Autodesk Inventor part; units mm, degrees
(part 2 of 3)
  line L635 (-116.0152, 0.9815) -> (-115.9907, 0.6998)
  line L636 (-115.9907, 0.6998) -> (-115.9907, 0.6019)
  line L637 (-115.9907, 0.6019) -> (-116.1009, 0.4794)
  line L638 (-116.1009, 0.4794) -> (-116.2968, -0.4267)
  spline S120 degree 2 poles (-116.2968, -0.4267) (-116.4682, -0.7573) (-116.4805, -0.7818) knots 0 0 0 1 1 1
  line L639 (-116.4805, -0.7818) -> (-116.4438, -0.892)
  line L640 (-116.4438, -0.892) -> (-116.4438, -0.99)
  spline S121 degree 2 poles (-116.4438, -0.99) (-116.5785, -1.3083) (-116.5785, -1.4553) knots 0 0 0 1 1 1
  line L641 (-116.5785, -1.4553) -> (-116.5785, -1.6267)
  line L642 (-116.5785, -1.6267) -> (-116.6519, -1.7002)
  line L643 (-116.6519, -1.7002) -> (-116.6274, -1.9083)
  line L644 (-116.6274, -1.9083) -> (-116.6887, -1.9451)
  line L645 (-116.6887, -1.9451) -> (-116.6519, -2.092)
  line L646 (-116.6519, -2.092) -> (-116.6887, -2.1287)
  line L647 (-116.6887, -2.1287) -> (-116.6887, -2.043)
  line L648 (-116.6887, -2.043) -> (-116.7621, -2.2879)
  spline S122 degree 2 poles (-116.7621, -2.2879) (-116.8356, -2.6185) (-116.958, -2.9736) (-117.154, -3.1818) knots 0 0 0 1 2 2 2
  line L649 (-117.154, -3.1818) -> (-117.1907, -3.3165)
  line L650 (-117.1907, -3.3165) -> (-117.2519, -3.3165)
  line L651 (-117.2519, -3.3165) -> (-117.3009, -3.4267)
  line L652 (-117.3009, -3.4267) -> (-117.2519, -3.4634)
  line L653 (-117.2519, -3.4634) -> (-117.3499, -3.5369)
  line L654 (-117.3499, -3.5369) -> (-117.3254, -3.5981)
  line L655 (-117.3254, -3.5981) -> (-117.4968, -3.9287)
  line L656 (-117.4968, -3.9287) -> (-117.5336, -4.0389)
  spline S123 degree 2 poles (-117.5336, -4.0389) (-117.5458, -4.1002) (-117.7785, -4.3818) knots 0 0 0 1 1 1
  line L657 (-117.7785, -4.3818) -> (-117.7785, -4.5165)
  line L658 (-117.7785, -4.5165) -> (-117.8274, -4.4553)
  spline S124 degree 2 poles (-117.8274, -4.4553) (-118.0111, -4.6757) (-118.1091, -4.7002) knots 0 0 0 1 1 1
  line L659 (-118.1091, -4.7002) -> (-118.1091, -4.9818)
  line L660 (-118.1091, -4.9818) -> (-118.3785, -5.4838)
  line L661 (-118.3785, -5.4838) -> (-118.4887, -5.4349)
  spline S125 degree 2 poles (-118.4887, -5.4349) (-118.5744, -5.6308) (-118.7703, -5.9614) knots 0 0 0 1 1 1
  line L662 (-118.7703, -5.9614) -> (-118.9295, -6.1328)
  spline S126 degree 2 poles (-118.9295, -6.1328) (-118.9785, -6.1818) (-119.1131, -6.4879) knots 0 0 0 1 1 1
  line L663 (-119.1131, -6.4879) -> (-119.3948, -6.6104)
  line L664 (-119.3948, -6.6104) -> (-119.3948, -6.6961)
  line L665 (-119.3948, -6.6961) -> (-119.456, -6.7818)
  line L666 (-119.456, -6.7818) -> (-119.5295, -6.7206)
  line L667 (-119.5295, -6.7206) -> (-119.7499, -7.1124)
  line L668 (-119.7499, -7.1124) -> (-119.9336, -7.0022)
  line L669 (-119.9336, -7.0022) -> (-120.1417, -7.2104)
  line L670 (-120.1417, -7.2104) -> (-120.1417, -7.1736)
  line L671 (-120.1417, -7.1736) -> (-120.2152, -7.2838)
  line L672 (-120.2152, -7.2838) -> (-120.2764, -7.2838)
  line L673 (-120.2764, -7.2838) -> (-120.3254, -7.3573)
  line L674 (-120.3254, -7.3573) -> (-120.3866, -7.3941)
  line L675 (-120.3866, -7.3941) -> (-120.4356, -7.492)
  line L676 (-120.4356, -7.492) -> (-120.4968, -7.4675)
  line L677 (-120.4968, -7.4675) -> (-120.607, -7.6145)
  line L678 (-120.607, -7.6145) -> (-120.7417, -7.6145)
  line L679 (-120.7417, -7.6145) -> (-120.8274, -7.7492)
  line L680 (-120.8274, -7.7492) -> (-120.9866, -7.7492)
  line L681 (-120.9866, -7.7492) -> (-121.1336, -7.7369)
  line L682 (-121.1336, -7.7369) -> (-121.2315, -7.6512)
  spline S127 degree 2 poles (-121.2315, -7.6512) (-121.2682, -7.6145) (-121.354, -7.3941) knots 0 0 0 1 1 1
  line L683 (-121.354, -7.3941) -> (-121.1948, -7.1369)
  line L684 (-121.1948, -7.1369) -> (-120.9621, -7.0389)
  line L685 (-120.9621, -7.0389) -> (-120.8519, -6.8553)
  line L686 (-120.8519, -6.8553) -> (-120.5703, -6.8308)
  line L687 (-120.5703, -6.8308) -> (-120.4968, -6.6471)
  line L688 (-120.4968, -6.6471) -> (-120.2764, -6.6104)
  line L689 (-120.2764, -6.6104) -> (-120.1172, -6.4389)
  spline S128 degree 2 poles (-120.1172, -6.4389) (-120.0438, -6.3655) (-119.6887, -6.1573) knots 0 0 0 1 1 1
  line L690 (-119.6887, -6.1573) -> (-119.6397, -5.8634)
  line L691 (-102.9131, 8.4998) -> (-102.6805, 8.2182)
  spline S129 degree 2 poles (-102.6805, 8.2182) (-102.8519, 7.8876) (-102.9621, 7.6182) knots 0 0 0 1 1 1
  line L692 (-102.9621, 7.6182) -> (-103.2315, 7.4468)
  line L693 (-103.2315, 7.4468) -> (-103.2927, 7.2753)
  line L694 (-103.2927, 7.2753) -> (-103.2315, 7.2264)
  line L695 (-103.2315, 7.2264) -> (-103.2315, 7.0917)
  line L696 (-103.2315, 7.0917) -> (-103.207, 7.0304)
  line L697 (-103.207, 7.0304) -> (-103.2682, 6.9447)
  line L698 (-103.2682, 6.9447) -> (-103.2682, 6.7855)
  line L699 (-103.2682, 6.7855) -> (-103.3785, 6.5284)
  line L700 (-103.3785, 6.5284) -> (-103.4764, 6.4549)
  spline S130 degree 2 poles (-103.4764, 6.4549) (-103.5989, 6.1243) (-103.6601, 5.8917) knots 0 0 0 1 1 1
  line L701 (-103.6601, 5.8917) -> (-103.8193, 5.757)
  line L702 (-103.8193, 5.757) -> (-103.8805, 5.5121)
  line L703 (-103.8805, 5.5121) -> (-103.8193, 5.4753)
  line L704 (-103.8193, 5.4753) -> (-104.0152, 5.2549)
  line L705 (-104.0152, 5.2549) -> (-104.0152, 5.0957)
  line L706 (-104.0152, 5.0957) -> (-104.0764, 5.01)
  line L707 (-104.0764, 5.01) -> (-103.9785, 4.5937)
  line L708 (-103.9785, 4.5937) -> (-104.0764, 4.2386)
  line L709 (-104.0764, 4.2386) -> (-104.0152, 3.81)
  line L710 (-104.0152, 3.81) -> (-103.9295, 3.5039)
  line L711 (-103.9295, 3.5039) -> (-103.9295, 3.2223)
  line L712 (-103.9295, 3.2223) -> (-103.8805, 2.8672)
  line L713 (-103.8805, 2.8672) -> (-103.9295, 2.7202)
  line L714 (-103.9295, 2.7202) -> (-103.9295, 2.3039)
  spline S131 degree 2 poles (-103.9295, 2.3039) (-103.7213, 2.4019) (-103.6234, 2.5121) knots 0 0 0 1 1 1
  line L715 (-103.6234, 2.5121) -> (-103.4764, 2.4753)
  line L716 (-103.4764, 2.4753) -> (-103.4764, 2.5855)
  line L717 (-103.4764, 2.5855) -> (-103.1213, 2.9284)
  line L718 (-103.1213, 2.9284) -> (-102.9621, 3.0386)
  line L719 (-102.9621, 3.0386) -> (-102.9621, 3.1121)
  line L720 (-102.9621, 3.1121) -> (-102.6805, 3.357)
  line L721 (-102.6805, 3.357) -> (-102.5948, 3.6141)
  spline S132 degree 2 poles (-102.5948, 3.6141) (-102.4234, 3.6998) (-102.3131, 3.81) knots 0 0 0 1 1 1
  line L722 (-102.3131, 3.81) -> (-102.2887, 3.7611)
  line L723 (-102.2887, 3.7611) -> (-102.2887, 3.8957)
  line L724 (-102.2887, 3.8957) -> (-102.1295, 4.0304)
  line L725 (-102.1295, 4.0304) -> (-102.1295, 3.957)
  line L726 (-102.1295, 3.957) -> (-102.0682, 4.0549)
  line L727 (-102.0682, 4.0549) -> (-101.958, 4.0549)
  line L728 (-101.958, 4.0549) -> (-101.958, 4.1406)
  line L729 (-101.958, 4.1406) -> (-101.9336, 4.2019)
  line L730 (-101.9336, 4.2019) -> (-101.7866, 4.2019)
  line L731 (-101.7866, 4.2019) -> (-101.7621, 4.3121)
  line L732 (-101.7621, 4.3121) -> (-101.7866, 4.4835)
  line L733 (-101.7866, 4.4835) -> (-101.2601, 4.9121)
  spline S133 degree 2 poles (-101.2601, 4.9121) (-101.1866, 4.9733) (-101.1621, 5.0468) knots 0 0 0 1 1 1
  line L734 (-101.1621, 5.0468) -> (-101.0764, 5.2304)
  spline S134 degree 2 poles (-101.0764, 5.2304) (-100.9295, 5.3162) (-100.7948, 5.3284) knots 0 0 0 1 1 1
  line L735 (-100.7948, 5.3284) -> (-100.758, 5.4508)
  line L736 (-100.758, 5.4508) -> (-100.6846, 5.5121)
  line L737 (-100.6846, 5.5121) -> (-100.5866, 5.5121)
  line L738 (-100.5866, 5.5121) -> (-100.5866, 5.6468)
  line L739 (-100.5866, 5.6468) -> (-100.5499, 5.5366)
  line L740 (-100.5499, 5.5366) -> (-100.5499, 5.6713)
  spline S135 degree 2 poles (-100.5499, 5.6713) (-100.4764, 5.8059) (-100.4029, 5.8304) knots 0 0 0 1 1 1
  line L741 (-100.4029, 5.8304) -> (-100.3785, 5.9284)
  line L742 (-100.3785, 5.9284) -> (-100.0234, 6.308)
  line L743 (-100.0234, 6.308) -> (-99.8764, 6.308)
  line L744 (-99.8764, 6.308) -> (-99.7417, 6.4549)
  line L745 (-99.7417, 6.4549) -> (-99.5948, 6.7488)
  spline S136 degree 2 poles (-99.5948, 6.7488) (-99.2274, 7.1529) (-99.1785, 7.2753) knots 0 0 0 1 1 1
  line L746 (-99.1785, 7.2753) -> (-98.958, 7.3121)
  line L747 (-98.958, 7.3121) -> (-98.7621, 7.6672)
  line L748 (-98.7621, 7.6672) -> (-98.8234, 7.4835)
  line L749 (-98.8234, 7.4835) -> (-98.5417, 7.7039)
  line L750 (-98.5417, 7.7039) -> (-98.3703, 7.5815)
  line L751 (-98.3703, 7.5815) -> (-98.1499, 7.7284)
  line L752 (-98.1499, 7.7284) -> (-97.8682, 7.7284)
  line L753 (-97.8682, 7.7284) -> (-97.7336, 7.6182)
  line L754 (-97.7336, 7.6182) -> (-97.6846, 7.3488)
  line L755 (-97.6846, 7.3488) -> (-97.807, 7.2264)
  spline S137 degree 2 poles (-97.807, 7.2264) (-97.8682, 7.1651) (-97.9785, 6.9202) knots 0 0 0 1 1 1
  line L756 (-97.9785, 6.9202) -> (-97.9295, 6.7855)
  line L757 (-97.9295, 6.7855) -> (-98.0152, 6.5284)
  line L758 (-98.0152, 6.5284) -> (-98.0152, 6.4304)
  line L759 (-98.0152, 6.4304) -> (-98.1254, 6.308)
  line L760 (-98.1254, 6.308) -> (-98.1254, 6.1121)
  line L761 (-98.1254, 6.1121) -> (-98.2601, 6.0753)
  line L762 (-98.2601, 6.0753) -> (-98.2601, 5.6713)
  line L763 (-98.2601, 5.6713) -> (-98.2846, 5.5121)
  line L764 (-98.2846, 5.5121) -> (-98.2601, 5.3284)
  line L765 (-98.2601, 5.3284) -> (-98.407, 5.1937)
  line L766 (-98.407, 5.1937) -> (-98.3213, 5.01)
  line L767 (-98.3213, 5.01) -> (-98.407, 4.8753)
  line L768 (-98.407, 4.8753) -> (-98.3213, 4.5325)
  line L769 (-98.3213, 4.5325) -> (-98.407, 4.3366)
  line L770 (-98.407, 4.3366) -> (-98.407, 3.0019)
  line L771 (-98.407, 3.0019) -> (-98.3213, 2.7202)
  line L772 (-98.3213, 2.7202) -> (-98.1866, 2.6223)
  line L773 (-98.1866, 2.6223) -> (-97.905, 2.6468)
  line L774 (-97.905, 2.6468) -> (-97.7703, 2.5121)
  line L775 (-97.7703, 2.5121) -> (-97.7948, 2.3406)
  line L776 (-97.7948, 2.3406) -> (-97.9785, 2.2549)
  line L777 (-97.9785, 2.2549) -> (-98.0519, 2.0835)
  line L778 (-98.0519, 2.0835) -> (-98.1866, 2.059)
  line L779 (-98.1866, 2.059) -> (-98.2846, 1.8753)
  line L780 (-98.2846, 1.8753) -> (-98.407, 1.8753)
  line L781 (-98.407, 1.8753) -> (-98.4682, 1.7039)
  line L782 (-98.4682, 1.7039) -> (-98.7866, 1.5937)
  line L783 (-98.7866, 1.5937) -> (-98.8968, 1.3855)
  line L784 (-98.8968, 1.3855) -> (-99.3254, 1.3121)
  line L785 (-99.3254, 1.3121) -> (-99.4846, 1.1406)
  line L786 (-99.4846, 1.1406) -> (-99.8397, 1.0672)
  line L787 (-99.8397, 1.0672) -> (-100.0234, 1.1774)
  line L788 (-100.0234, 1.1774) -> (-100.158, 1.6182)
  line L789 (-100.158, 1.6182) -> (-100.0234, 1.8141)
  line L790 (-100.0234, 1.8141) -> (-100.0968, 1.9488)
  line L791 (-100.0968, 1.9488) -> (-99.9866, 2.0835)
  line L792 (-99.9866, 2.0835) -> (-99.8397, 2.1202)
  line L793 (-99.8397, 2.1202) -> (-99.6805, 3.1733)
  line L794 (-99.6805, 3.1733) -> (-99.6805, 3.3202)
  line L795 (-99.6805, 3.3202) -> (-99.7662, 3.5039)
  line L796 (-99.7662, 3.5039) -> (-99.6315, 3.5651)
  line L797 (-99.6315, 3.5651) -> (-99.6805, 3.6998)
  line L798 (-99.6805, 3.6998) -> (-99.6315, 3.8957)
  line L799 (-99.6315, 3.8957) -> (-99.7662, 3.957)
  line L800 (-99.7662, 3.957) -> (-99.8397, 4.0549)
  line L801 (-99.8397, 4.0549) -> (-99.705, 4.1774)
  line L802 (-99.705, 4.1774) -> (-99.705, 4.3366)
  line L803 (-99.705, 4.3366) -> (-99.6315, 4.5325)
  spline S138 degree 2 poles (-99.6315, 4.5325) (-99.8274, 4.6917) (-99.9009, 4.6917) knots 0 0 0 1 1 1
  line L804 (-99.9009, 4.6917) -> (-99.9499, 5.059)
  line L805 (-99.9499, 5.059) -> (-100.0968, 5.059)
  line L806 (-100.0968, 5.059) -> (-100.207, 5.1202)
  line L807 (-100.207, 5.1202) -> (-100.3417, 4.8753)
  line L808 (-100.3417, 4.8753) -> (-101.1254, 4.0304)
  line L809 (-101.1254, 4.0304) -> (-101.2601, 3.9202)
  line L810 (-101.2601, 3.9202) -> (-101.2968, 3.81)
  line L811 (-101.2968, 3.81) -> (-101.8968, 3.1121)
  line L812 (-101.8968, 3.1121) -> (-101.958, 2.9774)
  line L813 (-101.958, 2.9774) -> (-102.5948, 2.2304)
  line L814 (-102.5948, 2.2304) -> (-103.3785, 1.3855)
  line L815 (-103.3785, 1.3855) -> (-103.6111, 1.2631)
  spline S139 degree 2 poles (-103.6111, 1.2631) (-103.6601, 1.2386) (-103.758, 1.0672) knots 0 0 0 1 1 1
  spline S140 degree 2 poles (-103.758, 1.0672) (-104.0887, 0.9447) (-104.1131, 0.9202) knots 0 0 0 1 1 1
  line L816 (-104.1131, 0.9202) -> (-104.1131, 0.8468)
  line L817 (-104.1131, 0.8468) -> (-104.2111, 0.8957)
  line L818 (-104.2111, 0.8957) -> (-104.2111, 0.6753)
  line L819 (-104.2111, 0.6753) -> (-104.4315, 0.5406)
  line L820 (-104.4315, 0.5406) -> (-104.7131, 0.5651)
  line L821 (-104.7131, 0.5651) -> (-104.9948, 0.3692)
  line L822 (-104.9948, 0.3692) -> (-105.0315, 0.4672)
  line L823 (-105.0315, 0.4672) -> (-105.2152, 0.5651)
  line L824 (-105.2152, 0.5651) -> (-105.2397, 0.7488)
  spline S141 degree 2 poles (-105.2397, 0.7488) (-105.3499, 0.8345) (-105.4234, 1.0059) knots 0 0 0 1 1 1
  line L825 (-105.4234, 1.0059) -> (-105.5948, 1.0672)
  line L826 (-105.5948, 1.0672) -> (-105.656, 1.2386)
  line L827 (-105.656, 1.2386) -> (-105.7662, 2.4508)
  line L828 (-105.7662, 2.4508) -> (-105.656, 2.9039)
  line L829 (-105.656, 2.9039) -> (-105.5948, 2.9039)
  line L830 (-105.5948, 2.9039) -> (-105.5948, 3.2223)
  line L831 (-105.5948, 3.2223) -> (-105.4234, 3.357)
  line L832 (-105.4234, 3.357) -> (-105.4478, 3.5039)
  line L833 (-105.4478, 3.5039) -> (-105.3499, 3.7611)
  line L834 (-105.3499, 3.7611) -> (-105.2152, 3.7611)
  line L835 (-105.2152, 3.7611) -> (-105.1785, 3.8468)
  line L836 (-105.1785, 3.8468) -> (-105.2152, 4.0549)
  line L837 (-105.2152, 4.0549) -> (-105.0927, 4.0917)
  line L838 (-105.0927, 4.0917) -> (-105.0682, 4.3366)
  line L839 (-105.0682, 4.3366) -> (-105.0315, 4.3733)
  line L840 (-105.0315, 4.3733) -> (-105.1295, 4.4835)
  line L841 (-105.1295, 4.4835) -> (-105.0315, 4.6917)
  line L842 (-105.0315, 4.6917) -> (-105.0315, 4.9488)
  line L843 (-105.0315, 4.9488) -> (-104.9948, 5.4753)
  line L844 (-104.9948, 5.4753) -> (-104.9336, 5.4753)
  line L845 (-104.9336, 5.4753) -> (-104.9336, 5.7325)
  line L846 (-104.9336, 5.7325) -> (-104.7866, 5.8917)
  line L847 (-104.7866, 5.8917) -> (-104.8968, 6.0386)
  line L848 (-104.8968, 6.0386) -> (-104.7866, 6.2223)
  line L849 (-104.7866, 6.2223) -> (-104.8234, 6.308)
  line L850 (-104.8234, 6.308) -> (-104.6764, 6.5896)
  line L851 (-104.6764, 6.5896) -> (-104.8968, 6.8468)
  line L852 (-104.8968, 6.8468) -> (-105.0315, 6.81)
  line L853 (-105.0315, 6.81) -> (-105.0682, 6.6753)
  line L854 (-105.0682, 6.6753) -> (-105.2764, 6.6386)
  line L855 (-105.2764, 6.6386) -> (-105.3499, 6.4549)
  line L856 (-105.3499, 6.4549) -> (-105.5948, 6.4549)
  line L857 (-105.5948, 6.4549) -> (-105.705, 6.5896)
  line L858 (-105.705, 6.5896) -> (-106.5499, 6.308)
  line L859 (-106.5499, 6.308) -> (-106.7703, 6.6753)
  line L860 (-106.7703, 6.6753) -> (-106.4887, 6.9447)
  spline S142 degree 2 poles (-106.4887, 6.9447) (-106.2682, 7.0427) (-106.207, 7.2264) knots 0 0 0 1 1 1
  line L861 (-106.207, 7.2264) -> (-105.9499, 7.2753)
  line L862 (-105.9499, 7.2753) -> (-105.9499, 7.3488)
  line L863 (-105.9499, 7.3488) -> (-105.7295, 7.3488)
  line L864 (-105.7295, 7.3488) -> (-105.4478, 7.3733)
  line L865 (-105.4478, 7.3733) -> (-105.2764, 7.7039)
  line L866 (-105.2764, 7.7039) -> (-104.9948, 7.6182)
  line L867 (-104.9948, 7.6182) -> (-104.6764, 7.7039)
  spline S143 degree 2 poles (-104.6764, 7.7039) (-104.6519, 7.7651) (-104.5785, 7.8264) knots 0 0 0 1 1 1
  line L868 (-104.5785, 7.8264) -> (-104.3213, 7.8264)
  line L869 (-104.3213, 7.8264) -> (-104.358, 7.8631)
  line L870 (-104.358, 7.8631) -> (-104.2968, 7.8998)
  line L871 (-104.2968, 7.8998) -> (-104.1131, 7.8998)
  line L872 (-104.1131, 7.8998) -> (-104.0764, 7.9855)
  spline S144 degree 2 poles (-104.0764, 7.9855) (-103.905, 8.0468) (-103.7336, 8.2182) knots 0 0 0 1 1 1
  line L873 (-103.7336, 8.2182) -> (-103.5989, 8.2182)
  line L874 (-103.5989, 8.2182) -> (-103.4764, 8.3651)
  line L875 (-103.4764, 8.3651) -> (-103.3785, 8.4019)
  line L876 (-103.3785, 8.4019) -> (-103.2682, 8.3651)
  line L877 (-103.2682, 8.3651) -> (-103.1213, 8.4386)
  line L878 (-103.1213, 8.4386) -> (-103.0478, 8.3651)
  line L879 (-103.0478, 8.3651) -> (-102.9866, 8.4998)
  line L880 (-102.9866, 8.4998) -> (-102.9131, 8.4998)
  line L881 (-83.9825, 12.81) -> (-83.9213, 12.7733)
  line L882 (-83.9213, 12.7733) -> (-83.7499, 12.7733)
  line L883 (-83.7499, 12.7733) -> (-83.0519, 12.2835)
  line L884 (-83.0519, 12.2835) -> (-82.5499, 11.757)
  line L885 (-82.5499, 11.757) -> (-83.3825, 11.1447)
  line L886 (-83.3825, 11.1447) -> (-83.4927, 11.01)
  line L887 (-83.4927, 11.01) -> (-84.0682, 10.8753)
  line L888 (-84.0682, 10.8753) -> (-84.3499, 10.8998)
  line L889 (-84.3499, 10.8998) -> (-84.5948, 11.0835)
  line L890 (-84.5948, 11.0835) -> (-84.7417, 11.0835)
  line L891 (-84.7417, 11.0835) -> (-85.3785, 9.7855)
  line L892 (-85.3785, 9.7855) -> (-85.6601, 9.4549)
  line L893 (-85.6601, 9.4549) -> (-85.6846, 9.1121)
  line L894 (-85.6846, 9.1121) -> (-85.9295, 8.6468)
  line L895 (-85.9295, 8.6468) -> (-86.0397, 8.2917)
  line L896 (-86.0397, 8.2917) -> (-86.1744, 8.0835)
  line L897 (-86.1744, 8.0835) -> (-86.2356, 7.5815)
  line L898 (-86.2356, 7.5815) -> (-86.3336, 7.3243)
  spline S145 degree 2 poles (-86.3336, 7.3243) (-86.358, 7.2753) (-86.5417, 7.0917) knots 0 0 0 1 1 1
  line L899 (-86.5417, 7.0917) -> (-86.5417, 6.9202)
  line L900 (-86.5417, 6.9202) -> (-86.6397, 6.5896)
  line L901 (-86.6397, 6.5896) -> (-86.5662, 6.3937)
  spline S146 degree 2 poles (-86.5662, 6.3937) (-86.6764, 6.0386) (-86.7744, 5.8917) knots 0 0 0 1 1 1
  line L902 (-86.7744, 5.8917) -> (-86.7376, 5.61)
  line L903 (-86.7376, 5.61) -> (-86.8478, 5.2549)
  line L904 (-86.8478, 5.2549) -> (-86.7744, 5.1937)
  line L905 (-86.7744, 5.1937) -> (-86.7744, 5.01)
  line L906 (-86.7744, 5.01) -> (-86.6397, 4.8753)
  line L907 (-86.6397, 4.8753) -> (-86.7131, 4.6182)
  line L908 (-86.7131, 4.6182) -> (-86.6397, 4.0549)
  line L909 (-86.6397, 4.0549) -> (-86.6764, 4.0549)
  line L910 (-86.6764, 4.0549) -> (-86.7131, 3.6386)
  spline S147 degree 2 poles (-86.7131, 3.6386) (-86.7131, 3.5162) (-86.3825, 3.1488) knots 0 0 0 1 1 1
  line L911 (-86.3825, 3.1488) -> (-86.456, 3.0386)
  line L912 (-86.456, 3.0386) -> (-86.3213, 2.8672)
  line L913 (-86.3213, 2.8672) -> (-86.2356, 2.157)
  line L914 (-86.2356, 2.157) -> (-86.4315, 1.9855)
  line L915 (-86.4315, 1.9855) -> (-86.4315, 1.7774)
  line L916 (-86.4315, 1.7774) -> (-86.5417, 1.5325)
  line L917 (-86.5417, 1.5325) -> (-86.6397, 1.5325)
  line L918 (-86.6397, 1.5325) -> (-86.958, 1.0672)
  line L919 (-86.958, 1.0672) -> (-87.2397, 1.0917)
  line L920 (-87.2397, 1.0917) -> (-87.4846, 0.7978)
  line L921 (-87.4846, 0.7978) -> (-87.9376, 0.4672)
  line L922 (-87.9376, 0.4672) -> (-88.2682, 1.0672)
  line L923 (-88.2682, 1.0672) -> (-88.2682, 1.6672)
  line L924 (-88.2682, 1.6672) -> (-88.3662, 2.2059)
  line L925 (-88.3662, 2.2059) -> (-88.3295, 2.4508)
  line L926 (-88.3295, 2.4508) -> (-88.758, 3.0753)
  line L927 (-88.758, 3.0753) -> (-88.6478, 3.259)
  line L928 (-88.6478, 3.259) -> (-88.758, 3.4549)
  line L929 (-88.758, 3.4549) -> (-88.6846, 3.5406)
  line L930 (-88.6846, 3.5406) -> (-88.9662, 3.6386)
  line L931 (-88.9662, 3.6386) -> (-89.0642, 3.5651)
  spline S148 degree 2 poles (-89.0642, 3.5651) (-89.1131, 3.6998) (-89.3458, 3.9692) knots 0 0 0 1 1 1
  line L932 (-89.3458, 3.9692) -> (-89.456, 3.9692)
  line L933 (-89.456, 3.9692) -> (-89.6274, 4.557)
  line L934 (-89.6274, 4.557) -> (-89.958, 4.8508)
  line L935 (-89.958, 4.8508) -> (-90.1295, 5.1937)
  spline S149 degree 2 poles (-90.1295, 5.1937) (-90.2519, 5.4141) (-90.2642, 5.5488) knots 0 0 0 1 1 1
  line L936 (-90.2642, 5.5488) -> (-90.6805, 5.9406)
  line L937 (-90.6805, 5.9406) -> (-90.7907, 6.1611)
  line L938 (-90.7907, 6.1611) -> (-90.7662, 6.3325)
  line L939 (-90.7662, 6.3325) -> (-90.8764, 6.5039)
  line L940 (-90.8764, 6.5039) -> (-90.9866, 6.5529)
  line L941 (-90.9866, 6.5529) -> (-91.0723, 6.7855)
  line L942 (-91.0723, 6.7855) -> (-91.158, 6.7855)
  line L943 (-91.158, 6.7855) -> (-91.2682, 7.0794)
  line L944 (-91.2682, 7.0794) -> (-91.4887, 7.3611)
  spline S150 degree 2 poles (-91.4887, 7.3611) (-91.5254, 7.4223) (-91.5744, 7.6427) knots 0 0 0 1 1 1
  line L945 (-91.5744, 7.6427) -> (-91.758, 7.6059)
  line L946 (-91.758, 7.6059) -> (-91.9662, 7.1651)
  line L947 (-91.9662, 7.1651) -> (-91.9662, 7.0304)
  spline S151 degree 2 poles (-91.9662, 7.0304) (-92.0152, 6.7243) (-92.1376, 6.3692) knots 0 0 0 1 1 1
  line L948 (-92.1376, 6.3692) -> (-92.2846, 6.2835)
  line L949 (-92.2846, 6.2835) -> (-92.2111, 6.0386)
  line L950 (-92.2111, 6.0386) -> (-92.0397, 5.9284)
  line L951 (-92.0397, 5.9284) -> (-92.1009, 5.5855)
  line L952 (-92.1009, 5.5855) -> (-92.1009, 5.1937)
  line L953 (-92.1009, 5.1937) -> (-92.456, 4.7651)
  line L954 (-92.456, 4.7651) -> (-92.4315, 4.459)
  line L955 (-92.4315, 4.459) -> (-92.5172, 4.2386)
  line L956 (-92.5172, 4.2386) -> (-92.4315, 3.9937)
  line L957 (-92.4315, 3.9937) -> (-92.4927, 3.9202)
  line L958 (-92.4927, 3.9202) -> (-92.456, 3.6998)
  line L959 (-92.456, 3.6998) -> (-92.6029, 3.3937)
  line L960 (-92.6029, 3.3937) -> (-92.6029, 3.1733)
  line L961 (-92.6029, 3.1733) -> (-92.7376, 3.0019)
  line L962 (-92.7376, 3.0019) -> (-92.8478, 2.5366)
  line L963 (-92.8478, 2.5366) -> (-92.8478, 2.4019)
  line L964 (-92.8478, 2.4019) -> (-92.9091, 2.3406)
  line L965 (-92.9091, 2.3406) -> (-93.2642, 1.2386)
  line L966 (-93.2642, 1.2386) -> (-93.3744, 1.0304)
  line L967 (-93.3744, 1.0304) -> (-93.656, 0.8957)
  line L968 (-93.656, 0.8957) -> (-93.6193, 0.81)
  line L969 (-93.6193, 0.81) -> (-94.1825, 0.5651)
  line L970 (-94.1825, 0.5651) -> (-94.4642, 0.6386)
  line L971 (-94.4642, 0.6386) -> (-94.5376, 0.9202)
  line L972 (-94.5376, 0.9202) -> (-94.354, 1.1406)
  line L973 (-94.354, 1.1406) -> (-94.4397, 1.2386)
  line L974 (-94.4397, 1.2386) -> (-94.6478, 1.2386)
  line L975 (-94.6478, 1.2386) -> (-94.6478, 1.3121)
  line L976 (-94.6478, 1.3121) -> (-94.4029, 1.5325)
  line L977 (-94.4029, 1.5325) -> (-94.4642, 1.8141)
  line L978 (-94.4642, 1.8141) -> (-94.2193, 1.8753)
  line L979 (-94.2193, 1.8753) -> (-93.8764, 2.3406)
  line L980 (-93.8764, 2.3406) -> (-93.7662, 2.757)
  line L981 (-93.7662, 2.757) -> (-93.7662, 2.9284)
  line L982 (-93.7662, 2.9284) -> (-93.5948, 3.1121)
  line L983 (-93.5948, 3.1121) -> (-93.5948, 3.4304)
  line L984 (-93.5948, 3.4304) -> (-93.1295, 5.3284)
  line L985 (-93.1295, 5.3284) -> (-93.154, 5.4508)
  line L986 (-93.154, 5.4508) -> (-93.154, 5.757)
  line L987 (-93.154, 5.757) -> (-92.958, 6.0753)
  line L988 (-92.958, 6.0753) -> (-93.0193, 6.2835)
  line L989 (-93.0193, 6.2835) -> (-92.8478, 6.5651)
  line L990 (-92.8478, 6.5651) -> (-92.8233, 6.7488)
  line L991 (-92.8233, 6.7488) -> (-92.7376, 7.0304)
  line L992 (-92.7376, 7.0304) -> (-92.7744, 7.1651)
  line L993 (-92.7744, 7.1651) -> (-92.6642, 7.5815)
  line L994 (-92.6642, 7.5815) -> (-92.958, 8.3406)
  spline S152 degree 2 poles (-92.958, 8.3406) (-92.8846, 8.4386) (-92.7376, 8.5366) knots 0 0 0 1 1 1
  line L995 (-92.7376, 8.5366) -> (-92.8478, 8.9284)
  line L996 (-92.8478, 8.9284) -> (-92.7744, 9.1733)
  line L997 (-92.7744, 9.1733) -> (-92.6274, 9.1978)
  line L998 (-92.6274, 9.1978) -> (-92.6029, 9.4182)
  line L999 (-92.6029, 9.4182) -> (-93.2397, 9.4182)
  line L1000 (-93.2397, 9.4182) -> (-93.8764, 9.1978)
  line L1001 (-93.8764, 9.1978) -> (-94.0111, 9.2835)
  line L1002 (-94.0111, 9.2835) -> (-94.354, 8.5855)
  line L1003 (-94.354, 8.5855) -> (-95.2356, 7.7651)
  line L1004 (-95.2356, 7.7651) -> (-95.7131, 7.557)
  line L1005 (-95.7131, 7.557) -> (-95.9091, 7.9488)
  line L1006 (-95.9091, 7.9488) -> (-95.9091, 8.2182)
  line L1007 (-95.9091, 8.2182) -> (-95.7376, 8.2917)
  line L1008 (-95.7376, 8.2917) -> (-95.7744, 8.4386)
  line L1009 (-95.7744, 8.4386) -> (-95.8723, 8.4753)
  line L1010 (-95.8723, 8.4753) -> (-95.8723, 8.6468)
  line L1011 (-95.8723, 8.6468) -> (-95.7131, 8.7815)
  line L1012 (-95.7131, 8.7815) -> (-95.7131, 8.9284)
  line L1013 (-95.7131, 8.9284) -> (-95.4315, 8.8304)
  line L1014 (-95.4315, 8.8304) -> (-95.358, 8.9284)
  line L1015 (-95.358, 8.9284) -> (-95.456, 9.0386)
  spline S153 degree 2 poles (-95.456, 9.0386) (-95.4315, 9.1121) (-95.1376, 9.4549) knots 0 0 0 1 1 1
  line L1016 (-95.1376, 9.4549) -> (-94.7458, 9.5651)
  line L1017 (-94.7458, 9.5651) -> (-94.7213, 9.81)
  line L1018 (-94.7213, 9.81) -> (-94.5376, 9.7855)
  line L1019 (-94.5376, 9.7855) -> (-94.3907, 9.9447)
  spline S154 degree 2 poles (-94.3907, 9.9447) (-94.354, 9.9815) (-94.2315, 10.0304) knots 0 0 0 1 1 1
  line L1020 (-94.2315, 10.0304) -> (-93.9376, 10.1406)
  line L1021 (-93.9376, 10.1406) -> (-93.9009, 10.2019)
  line L1022 (-93.9009, 10.2019) -> (-93.6927, 10.2141)
  spline S155 degree 2 poles (-93.6927, 10.2141) (-93.558, 10.2386) (-93.3621, 10.3855) (-92.9948, 10.4468) knots 0 0 0 1 2 2 2
  line L1023 (-92.9948, 10.4468) -> (-92.6274, 10.508)
  line L1024 (-92.6274, 10.508) -> (-91.7825, 10.9978)
  line L1025 (-91.7825, 10.9978) -> (-91.5744, 11.2182)
  line L1026 (-91.5744, 11.2182) -> (-91.1458, 11.3774)
  line L1027 (-91.1458, 11.3774) -> (-90.7662, 11.4264)
  line L1028 (-90.7662, 11.4264) -> (-90.5703, 11.0223)
  spline S156 degree 2 poles (-90.5703, 11.0223) (-90.7907, 10.6427) (-90.7417, 10.459) knots 0 0 0 1 1 1
  line L1029 (-90.7417, 10.459) -> (-90.5213, 9.2345)
  line L1030 (-90.5213, 9.2345) -> (-90.4111, 8.9406)
  line L1031 (-90.4111, 8.9406) -> (-90.4111, 8.7447)
  line L1032 (-90.4111, 8.7447) -> (-90.2029, 8.7447)
  line L1033 (-90.2029, 8.7447) -> (-90.1785, 8.4264)
  line L1034 (-90.1785, 8.4264) -> (-89.8478, 8.1447)
  line L1035 (-89.8478, 8.1447) -> (-89.8846, 7.9488)
  line L1036 (-89.8846, 7.9488) -> (-89.8111, 7.8631)
  line L1037 (-89.8111, 7.8631) -> (-89.2111, 6.8468)
  line L1038 (-89.2111, 6.8468) -> (-88.5744, 5.5855)
  line L1039 (-88.5744, 5.5855) -> (-88.4029, 5.4019)
  line L1040 (-88.4029, 5.4019) -> (-88.4029, 5.3039)
  line L1041 (-88.4029, 5.3039) -> (-88.2682, 5.157)
  line L1042 (-88.2682, 5.157) -> (-88.0478, 5.1202)
  line L1043 (-88.0478, 5.1202) -> (-88.0111, 5.3039)
  line L1044 (-88.0111, 5.3039) -> (-87.9131, 5.3284)
  line L1045 (-87.9131, 5.3284) -> (-87.9131, 5.4508)
  line L1046 (-87.9131, 5.4508) -> (-87.6315, 6.3692)
  line L1047 (-87.6315, 6.3692) -> (-87.607, 6.5896)
  spline S157 degree 2 poles (-87.607, 6.5896) (-87.5948, 6.6753) (-87.4601, 7.0672) knots 0 0 0 1 1 1
  line L1048 (-87.4601, 7.0672) -> (-87.154, 7.2753)
  line L1049 (-87.154, 7.2753) -> (-87.154, 7.4468)
  line L1050 (-87.154, 7.4468) -> (-86.9948, 7.7284)
  line L1051 (-86.9948, 7.7284) -> (-86.9948, 7.9488)
  spline S158 degree 2 poles (-86.9948, 7.9488) (-86.8233, 8.157) (-86.7376, 8.4998) knots 0 0 0 1 1 1
  spline S159 degree 2 poles (-86.7376, 8.4998) (-86.6887, 8.5243) (-86.6152, 8.6223) knots 0 0 0 1 1 1
  line L1052 (-86.6152, 8.6223) -> (-86.5417, 8.7202)
  line L1053 (-86.5417, 8.7202) -> (-86.1009, 9.8835)
  spline S160 degree 2 poles (-86.1009, 9.8835) (-86.0274, 10.0549) (-85.954, 10.1039) knots 0 0 0 1 1 1
  line L1054 (-85.954, 10.1039) -> (-85.856, 10.508)
  line L1055 (-85.856, 10.508) -> (-85.7213, 10.6182)
  line L1056 (-85.7213, 10.6182) -> (-85.5376, 10.9488)
  line L1057 (-85.5376, 10.9488) -> (-85.4397, 11.2549)
  line L1058 (-85.4397, 11.2549) -> (-85.305, 11.4264)
  spline S161 degree 2 poles (-85.305, 11.4264) (-85.2315, 11.4998) (-85.158, 11.7202) knots 0 0 0 1 1 1
  line L1059 (-85.158, 11.7202) -> (-85.0233, 11.757)
  line L1060 (-85.0233, 11.757) -> (-84.6193, 12.4917)
  line L1061 (-84.6193, 12.4917) -> (-84.4601, 12.6386)
  line L1062 (-84.4601, 12.6386) -> (-84.3866, 12.6386)
  spline S162 degree 2 poles (-84.3866, 12.6386) (-84.2887, 12.7733) (-84.2397, 12.7733) knots 0 0 0 1 1 1
  line L1063 (-84.2397, 12.7733) -> (-83.9825, 12.81)
  line L1064 (-79.158, 8.2182) -> (-78.9744, 8.1937)
  line L1065 (-78.9744, 8.1937) -> (-78.9376, 8.1937)
  line L1066 (-78.9376, 8.1937) -> (-78.9744, 8.1202)
  line L1067 (-78.9744, 8.1202) -> (-78.9131, 8.1202)
  line L1068 (-78.9131, 8.1202) -> (-78.8029, 8.01)
  line L1069 (-78.8029, 8.01) -> (-78.4478, 7.9855)
  line L1070 (-78.4478, 7.9855) -> (-78.0927, 7.9855)
  line L1071 (-78.0927, 7.9855) -> (-77.8846, 7.8631)
  line L1072 (-77.8846, 7.8631) -> (-77.8111, 7.8631)
  line L1073 (-77.8111, 7.8631) -> (-77.7009, 7.4835)
  line L1074 (-77.7009, 7.4835) -> (-77.8601, 7.3488)
  line L1075 (-77.8601, 7.3488) -> (-77.8601, 7.2019)
  line L1076 (-77.8601, 7.2019) -> (-77.6029, 6.9447)
  line L1077 (-77.6029, 6.9447) -> (-77.6397, 6.2468)
  line L1078 (-77.6397, 6.2468) -> (-77.7499, 6.2468)
  line L1079 (-77.7499, 6.2468) -> (-77.7866, 6.1121)
  line L1080 (-77.7866, 6.1121) -> (-77.8111, 6.1121)
  line L1081 (-77.8111, 6.1121) -> (-77.8111, 5.8917)
  line L1082 (-77.8111, 5.8917) -> (-77.6642, 5.8672)
  line L1083 (-77.6642, 5.8672) -> (-77.6029, 5.7937)
  line L1084 (-77.6029, 5.7937) -> (-77.7009, 5.6468)
  line L1085 (-77.7009, 5.6468) -> (-77.7009, 5.5366)
  line L1086 (-77.7009, 5.5366) -> (-77.8846, 5.4508)
  line L1087 (-77.8846, 5.4508) -> (-78.0193, 5.3284)
  line L1088 (-78.0193, 5.3284) -> (-78.4233, 5.1202)
  spline S163 degree 2 poles (-78.4233, 5.1202) (-78.5825, 4.9488) (-78.6927, 4.8753) knots 0 0 0 1 1 1
  line L1089 (-78.6927, 4.8753) -> (-78.8029, 4.557)
  line L1090 (-78.8029, 4.557) -> (-79.4764, 4.2998)
  line L1091 (-79.4764, 4.2998) -> (-80.1376, 4.3121)
  line L1092 (-80.1376, 4.3121) -> (-80.1131, 4.1406)
  line L1093 (-80.1131, 4.1406) -> (-80.2478, 4.1406)
  line L1094 (-80.2478, 4.1406) -> (-80.2846, 4.0917)
  line L1095 (-80.2846, 4.0917) -> (-80.6029, 4.0304)
  line L1096 (-80.6029, 4.0304) -> (-80.6397, 4.1406)
  line L1097 (-80.6397, 4.1406) -> (-80.7499, 4.0917)
  line L1098 (-80.7499, 4.0917) -> (-80.7499, 4.0304)
  line L1099 (-80.7499, 4.0304) -> (-81.0315, 3.9202)
  line L1100 (-81.0315, 3.9202) -> (-81.1417, 3.6141)
  line L1101 (-81.1417, 3.6141) -> (-80.9948, 3.2223)
  line L1102 (-80.9948, 3.2223) -> (-80.9948, 3.0386)
  line L1103 (-80.9948, 3.0386) -> (-80.9213, 2.8672)
  spline S164 degree 2 poles (-80.9213, 2.8672) (-81.0682, 2.4141) (-81.1417, 2.4019) knots 0 0 0 1 1 1
  line L1104 (-81.1417, 2.4019) -> (-81.0927, 2.2549)
  line L1105 (-81.0927, 2.2549) -> (-81.1662, 2.2304)
  line L1106 (-81.1662, 2.2304) -> (-80.9948, 2.157)
  line L1107 (-80.9948, 2.157) -> (-80.9948, 1.9243)
  line L1108 (-80.9948, 1.9243) -> (-80.8356, 1.8141)
  spline S165 degree 2 poles (-80.8356, 1.8141) (-80.456, 1.9243) (-80.3825, 1.9855) knots 0 0 0 1 1 1
  line L1109 (-80.3825, 1.9855) -> (-80.2601, 1.8753)
  line L1110 (-80.2601, 1.8753) -> (-80.2356, 1.8998)
  spline S166 degree 2 poles (-80.2356, 1.8998) (-79.9172, 1.9366) (-79.7458, 1.9855) knots 0 0 0 1 1 1
  line L1111 (-79.7458, 1.9855) -> (-79.6846, 2.0713)
  line L1112 (-79.6846, 2.0713) -> (-79.5009, 2.0713)
  line L1113 (-79.5009, 2.0713) -> (-79.3662, 2.0835)
  line L1114 (-79.3662, 2.0835) -> (-79.1825, 1.9978)
  line L1115 (-79.1825, 1.9978) -> (-79.2193, 2.059)
  line L1116 (-79.2193, 2.059) -> (-79.0723, 2.059)
  line L1117 (-79.0723, 2.059) -> (-78.8887, 2.2182)
  line L1118 (-78.8887, 2.2182) -> (-78.6682, 2.2304)
  line L1119 (-78.6682, 2.2304) -> (-78.705, 2.2304)
  line L1120 (-78.705, 2.2304) -> (-78.4968, 2.3162)
  line L1121 (-78.4968, 2.3162) -> (-78.4356, 2.2794)
  line L1122 (-78.4356, 2.2794) -> (-78.3254, 2.3774)
  line L1123 (-78.3254, 2.3774) -> (-78.1662, 2.3774)
  line L1124 (-78.1662, 2.3774) -> (-78.0193, 2.5243)
  spline S167 degree 2 poles (-78.0193, 2.5243) (-77.8601, 2.5366) (-77.4805, 2.7202) knots 0 0 0 1 1 1
  line L1125 (-77.4805, 2.7202) -> (-77.4805, 2.8059)
  line L1126 (-77.4805, 2.8059) -> (-77.2723, 2.8672)
  line L1127 (-77.2723, 2.8672) -> (-77.0274, 3.21)
  line L1128 (-77.0274, 3.21) -> (-76.7825, 3.1733)
  spline S168 degree 2 poles (-76.7825, 3.1733) (-76.6478, 3.0631) (-76.4764, 3.0386) knots 0 0 0 1 1 1
  line L1129 (-76.4764, 3.0386) -> (-76.3662, 2.9284)
  line L1130 (-76.3662, 2.9284) -> (-76.5376, 2.5978)
  line L1131 (-76.5376, 2.5978) -> (-76.5131, 2.4019)
  line L1132 (-76.5131, 2.4019) -> (-76.7458, 2.2549)
  line L1133 (-76.7458, 2.2549) -> (-76.7825, 2.1815)
  line L1134 (-76.7825, 2.1815) -> (-77.1499, 2.1447)
  line L1135 (-77.1499, 2.1447) -> (-77.3458, 1.9366)
  line L1136 (-77.3458, 1.9366) -> (-77.5662, 1.9243)
  line L1137 (-77.5662, 1.9243) -> (-77.6274, 1.7406)
  line L1138 (-77.6274, 1.7406) -> (-77.9213, 1.7774)
  line L1139 (-77.9213, 1.7774) -> (-78.007, 1.557)
  line L1140 (-78.007, 1.557) -> (-78.2397, 1.5937)
  line L1141 (-78.2397, 1.5937) -> (-78.3376, 1.4835)
  spline S169 degree 2 poles (-78.3376, 1.4835) (-78.5948, 1.3855) (-78.607, 1.3733) knots 0 0 0 1 1 1
  line L1142 (-78.607, 1.3733) -> (-78.705, 1.4345)
  line L1143 (-78.705, 1.4345) -> (-78.8887, 1.2631)
  line L1144 (-78.8887, 1.2631) -> (-79.1336, 1.2631)
  line L1145 (-79.1336, 1.2631) -> (-79.2805, 1.1896)
  line L1146 (-79.2805, 1.1896) -> (-79.3785, 1.1896)
  line L1147 (-79.3785, 1.1896) -> (-79.4887, 1.0917)
  spline S170 degree 2 poles (-79.4887, 1.0917) (-79.6846, 1.0427) (-79.8927, 0.9202) knots 0 0 0 1 1 1
  line L1148 (-79.8927, 0.9202) -> (-80.0029, 1.0059)
  line L1149 (-80.0029, 1.0059) -> (-80.2233, 1.0059)
  line L1150 (-80.2233, 1.0059) -> (-80.3091, 0.9202)
  line L1151 (-80.3091, 0.9202) -> (-80.3948, 0.957)
  line L1152 (-80.3948, 0.957) -> (-80.4927, 0.9202)
  line L1153 (-80.4927, 0.9202) -> (-80.5295, 0.957)
  line L1154 (-80.5295, 0.957) -> (-80.6029, 0.7855)
  line L1155 (-80.6029, 0.7855) -> (-80.8111, 0.7855)
  line L1156 (-80.8111, 0.7855) -> (-80.9825, 0.6876)
  spline S171 degree 2 poles (-80.9825, 0.6876) (-81.056, 0.6386) (-81.3376, 0.6141) knots 0 0 0 1 1 1
  line L1157 (-81.3376, 0.6141) -> (-81.4111, 0.5406)
  line L1158 (-81.4111, 0.5406) -> (-81.558, 0.5406)
  line L1159 (-81.558, 0.5406) -> (-81.754, 0.5039)
  line L1160 (-81.754, 0.5039) -> (-81.9131, 0.3202)
  line L1161 (-81.9131, 0.3202) -> (-82.1091, 0.3937)
  line L1162 (-82.1091, 0.3937) -> (-82.2193, 0.259)
  line L1163 (-82.2193, 0.259) -> (-82.305, 0.2835)
  spline S172 degree 2 poles (-82.305, 0.2835) (-82.3295, 0.2835) (-82.6111, 0.5651) knots 0 0 0 1 1 1
  line L1164 (-82.6111, 0.5651) -> (-82.5744, 0.7488)
  line L1165 (-82.5744, 0.7488) -> (-82.6111, 0.8468)
  line L1166 (-82.6111, 0.8468) -> (-82.5744, 1.0304)
  line L1167 (-82.5744, 1.0304) -> (-82.6968, 1.3121)
  line L1168 (-82.6968, 1.3121) -> (-82.6478, 1.5325)
  line L1169 (-82.6478, 1.5325) -> (-82.7213, 1.8753)
  line L1170 (-82.7213, 1.8753) -> (-82.6478, 2.157)
  line L1171 (-82.6478, 2.157) -> (-82.758, 2.5855)
  line L1172 (-82.758, 2.5855) -> (-82.7825, 2.6223)
  line L1173 (-82.7825, 2.6223) -> (-82.758, 2.8427)
  line L1174 (-82.758, 2.8427) -> (-82.5009, 2.9284)
  line L1175 (-82.5009, 2.9284) -> (-82.5009, 3.0753)
  line L1176 (-82.5009, 3.0753) -> (-82.6111, 3.1121)
  line L1177 (-82.6111, 3.1121) -> (-82.5744, 3.3202)
  line L1178 (-82.5744, 3.3202) -> (-82.6478, 3.4304)
  line L1179 (-82.6478, 3.4304) -> (-82.6111, 3.6141)
  line L1180 (-82.6111, 3.6141) -> (-82.5009, 3.6753)
  line L1181 (-82.5009, 3.6753) -> (-82.5376, 3.8468)
  line L1182 (-82.5376, 3.8468) -> (-82.5009, 4.1406)
  line L1183 (-82.5009, 4.1406) -> (-82.4397, 4.1774)
  line L1184 (-82.4397, 4.1774) -> (-82.3295, 4.5325)
  line L1185 (-82.3295, 4.5325) -> (-82.0846, 4.9733)
  line L1186 (-82.0846, 4.9733) -> (-81.8642, 5.059)
  line L1187 (-81.8642, 5.059) -> (-81.8397, 5.3039)
  line L1188 (-81.8397, 5.3039) -> (-81.8642, 5.3774)
  line L1189 (-81.8642, 5.3774) -> (-81.8397, 5.5121)
  line L1190 (-81.8397, 5.5121) -> (-81.6927, 5.5855)
  line L1191 (-81.6927, 5.5855) -> (-81.6193, 5.8304)
  line L1192 (-81.6193, 5.8304) -> (-81.8029, 5.8304)
  line L1193 (-81.8029, 5.8304) -> (-81.8029, 5.9284)
  line L1194 (-81.8029, 5.9284) -> (-81.7295, 6.0386)
  line L1195 (-81.7295, 6.0386) -> (-81.754, 6.1488)
  line L1196 (-81.754, 6.1488) -> (-81.7295, 6.2468)
  line L1197 (-81.7295, 6.2468) -> (-81.6927, 6.2468)
  line L1198 (-81.6927, 6.2468) -> (-81.6927, 6.5039)
  line L1199 (-81.6927, 6.5039) -> (-81.4478, 6.5284)
  line L1200 (-81.4478, 6.5284) -> (-81.3376, 6.7488)
  line L1201 (-81.3376, 6.7488) -> (-80.8111, 7.3488)
  line L1202 (-80.8111, 7.3488) -> (-80.7009, 7.3488)
  spline S173 degree 2 poles (-80.7009, 7.3488) (-80.6152, 7.4835) (-80.4682, 7.5815) knots 0 0 0 1 1 1
  line L1203 (-80.4682, 7.5815) -> (-80.358, 7.557)
  spline S174 degree 2 poles (-80.358, 7.557) (-80.2601, 7.5937) (-80.1131, 7.8019) knots 0 0 0 1 1 1
  line L1204 (-80.1131, 7.8019) -> (-80.0397, 7.8019)
  line L1205 (-80.0397, 7.8019) -> (-79.8927, 7.8998)
  line L1206 (-79.8927, 7.8998) -> (-79.8315, 7.8998)
  line L1207 (-79.8315, 7.8998) -> (-79.7213, 8.059)
  line L1208 (-79.7213, 8.059) -> (-79.158, 8.2182)
  line L1209 (-79.3417, 6.9325) -> (-79.6111, 6.8468)
  line L1210 (-79.6111, 6.8468) -> (-79.8193, 6.9325)
  spline S175 degree 2 poles (-79.8193, 6.9325) (-80.0029, 6.7855) (-80.1131, 6.7243) knots 0 0 0 1 1 1
  spline S176 degree 2 poles (-80.1131, 6.7243) (-80.1376, 6.5284) (-80.3948, 6.2468) (-80.456, 6.2468) knots 0 0 0 1 2 2 2
  line L1211 (-80.456, 6.2468) -> (-80.5907, 6.2468)
  line L1212 (-80.5907, 6.2468) -> (-80.4927, 6.0876)
  spline S177 degree 2 poles (-80.4927, 6.0876) (-80.5785, 5.9284) (-80.7131, 5.61) knots 0 0 0 1 1 1
  line L1213 (-80.7131, 5.61) -> (-80.8356, 5.6468)
  line L1214 (-80.8356, 5.6468) -> (-80.8846, 5.4508)
  line L1215 (-80.8846, 5.4508) -> (-80.8356, 5.1692)
  line L1216 (-80.8356, 5.1692) -> (-80.6887, 5.0835)
  spline S178 degree 2 poles (-80.6887, 5.0835) (-80.6152, 5.0468) (-80.3091, 4.9978) knots 0 0 0 1 1 1
  line L1217 (-80.3091, 4.9978) -> (-80.0642, 5.157)
  line L1218 (-80.0642, 5.157) -> (-79.5621, 5.1937)
  line L1219 (-79.5621, 5.1937) -> (-79.305, 5.5855)
  line L1220 (-79.305, 5.5855) -> (-78.9376, 5.8794)
  line L1221 (-78.9376, 5.8794) -> (-78.9009, 6.4427)
  line L1222 (-78.9009, 6.4427) -> (-79.0233, 6.6264)
  line L1223 (-79.0233, 6.6264) -> (-79.0356, 6.8835)
  line L1224 (-79.0356, 6.8835) -> (-79.207, 6.8835)
  line L1225 (-79.207, 6.8835) -> (-79.3417, 6.9325)
  line L1226 (-72.5458, 7.3611) -> (-72.5703, 7.3611)
  line L1227 (-72.5703, 7.3611) -> (-72.6315, 6.9692)
  line L1228 (-72.6315, 6.9692) -> (-72.5703, 6.9202)
  line L1229 (-72.5703, 6.9202) -> (-72.6805, 6.6386)
  line L1230 (-72.6805, 6.6386) -> (-72.7172, 6.6876)
  line L1231 (-72.7172, 6.6876) -> (-72.7172, 6.5774)
  spline S179 degree 2 poles (-72.7172, 6.5774) (-72.7172, 6.2468) (-72.9866, 5.9406) knots 0 0 0 1 1 1
  line L1232 (-72.9866, 5.9406) -> (-72.9376, 5.9406)
  line L1233 (-72.9376, 5.9406) -> (-72.9376, 5.8059)
  line L1234 (-72.9376, 5.8059) -> (-72.9621, 5.8059)
  line L1235 (-72.9621, 5.8059) -> (-72.9376, 4.9121)
  line L1236 (-72.9376, 4.9121) -> (-72.9866, 4.8141)
  line L1237 (-72.9866, 4.8141) -> (-72.9621, 4.6672)
  line L1238 (-72.9621, 4.6672) -> (-73.0723, 4.1162)
  line L1239 (-73.0723, 4.1162) -> (-73.0356, 4.1162)
  spline S180 degree 2 poles (-73.0356, 4.1162) (-73.0356, 3.957) (-73.1091, 3.6753) knots 0 0 0 1 1 1
  line L1240 (-73.1091, 3.6753) -> (-73.1825, 3.4794)
  line L1241 (-73.1825, 3.4794) -> (-73.2682, 2.4631)
  spline S181 degree 2 poles (-73.2682, 2.4631) (-73.305, 2.3162) (-73.305, 2.2917) knots 0 0 0 1 1 1
  spline S182 degree 2 poles (-73.305, 2.2917) (-73.305, 2.157) (-73.1825, 2.157) knots 0 0 0 1 1 1
  spline S183 degree 2 poles (-73.1825, 2.157) (-73.0356, 2.157) (-72.8642, 2.2672) knots 0 0 0 1 1 1
  line L1242 (-72.8642, 2.2672) -> (-72.3744, 2.5978)
  spline S184 degree 2 poles (-72.3744, 2.5978) (-72.1662, 2.8549) (-72.0682, 2.8549) knots 0 0 0 1 1 1
  line L1243 (-72.0682, 2.8549) -> (-72.0315, 2.8549)
  spline S185 degree 2 poles (-72.0315, 2.8549) (-71.8968, 2.9162) (-71.6764, 3.1978) (-71.6152, 3.2223) knots 0 0 0 1 2 2 2
  spline S186 degree 2 poles (-71.6152, 3.2223) (-71.4927, 3.4304) (-71.407, 3.4304) knots 0 0 0 1 1 1
  spline S187 degree 2 poles (-71.407, 3.4304) (-71.3948, 3.4304) (-71.2968, 3.3937) (-71.0642, 3.357) knots 0 0 0 1 2 2 2
  line L1244 (-71.0642, 3.357) -> (-71.0029, 3.1488)
  spline S188 degree 2 poles (-71.0029, 3.1488) (-71.0029, 2.9774) (-71.2478, 2.5243) (-71.3948, 2.2304) (-71.6397, 2.1447) knots 0 0 0 1 2 3 3 3
  line L1245 (-71.6397, 2.1447) -> (-71.6397, 2.0835)
  line L1246 (-71.6397, 2.0835) -> (-71.7499, 2.1202)
  line L1247 (-71.7499, 2.1202) -> (-71.7499, 2.01)
  line L1248 (-71.7499, 2.01) -> (-71.8111, 2.01)
  spline S189 degree 2 poles (-71.8111, 2.01) (-71.8356, 1.8019) (-72.0315, 1.7774) knots 0 0 0 1 1 1
  line L1249 (-72.0315, 1.7774) -> (-72.0315, 1.7284)
  line L1250 (-72.0315, 1.7284) -> (-72.2397, 1.7284)
  line L1251 (-72.2397, 1.7284) -> (-72.2397, 1.7039)
  line L1252 (-72.2397, 1.7039) -> (-72.3131, 1.7039)
  line L1253 (-72.3131, 1.7039) -> (-72.5091, 1.557)
  line L1254 (-72.5091, 1.557) -> (-72.5703, 1.557)
  line L1255 (-72.5703, 1.557) -> (-72.6805, 1.4223)
  line L1256 (-72.6805, 1.4223) -> (-72.9866, 1.3733)
  spline S190 degree 2 poles (-72.9866, 1.3733) (-73.0356, 1.2876) (-73.1336, 1.2876) knots 0 0 0 1 1 1
  line L1257 (-73.1336, 1.2876) -> (-73.5254, 1.0059)
  line L1258 (-73.5254, 1.0059) -> (-73.5254, 0.9447)
  line L1259 (-73.5254, 0.9447) -> (-73.7091, 0.9692)
  line L1260 (-73.7091, 0.9692) -> (-73.6601, 0.8957)
  line L1261 (-73.6601, 0.8957) -> (-73.905, 0.8345)
  line L1262 (-73.905, 0.8345) -> (-73.905, 0.7978)
  line L1263 (-73.905, 0.7978) -> (-74.0152, 0.7978)
  line L1264 (-74.0152, 0.7978) -> (-74.0152, 0.6876)
  line L1265 (-74.0152, 0.6876) -> (-74.1254, 0.6141)
  line L1266 (-74.1254, 0.6141) -> (-74.1621, 0.6141)
  line L1267 (-74.1621, 0.6141) -> (-74.1621, 0.5896)
  spline S191 degree 2 poles (-74.1621, 0.5896) (-74.2601, 0.308) (-74.4438, 0.308) knots 0 0 0 1 1 1
  line L1268 (-74.4438, 0.308) -> (-74.5417, 0.3325)
  spline S192 degree 2 poles (-74.5417, 0.3325) (-74.6397, 0.6141) (-74.8601, 0.8957) knots 0 0 0 1 1 1
  spline S193 degree 2 poles (-74.8601, 0.8957) (-74.7989, 1.1406) (-74.7989, 1.2508) knots 0 0 0 1 1 1
  line L1269 (-74.7989, 1.2508) -> (-74.8601, 1.557)
  line L1270 (-74.8601, 1.557) -> (-74.8601, 1.7284)
  spline S194 degree 2 poles (-74.8601, 1.7284) (-74.8601, 1.9611) (-74.8111, 2.2182) knots 0 0 0 1 1 1
  line L1271 (-74.8111, 2.2182) -> (-74.7621, 2.4141)
  line L1272 (-74.7621, 2.4141) -> (-74.7621, 2.4508)
  line L1273 (-74.7621, 2.4508) -> (-74.7866, 2.4508)
  spline S195 degree 2 poles (-74.7866, 2.4508) (-74.7989, 2.4508) (-74.7989, 2.4631) knots 0 0 0 1 1 1
  spline S196 degree 2 poles (-74.7989, 2.4631) (-74.7989, 2.4753) (-74.6519, 2.9406) (-74.6519, 3.2957) knots 0 0 0 1 2 2 2
  spline S197 degree 2 poles (-74.6519, 3.2957) (-74.6519, 3.3937) (-74.7254, 3.4059) knots 0 0 0 1 1 1
  line L1274 (-74.7254, 3.4059) -> (-74.6274, 3.6141)
  line L1275 (-74.6274, 3.6141) -> (-74.6274, 4.5325)
  line L1276 (-74.6274, 4.5325) -> (-74.505, 4.7896)
  spline S198 degree 2 poles (-74.505, 4.7896) (-74.4438, 4.9121) (-74.3825, 5.2672) knots 0 0 0 1 1 1
  spline S199 degree 2 poles (-74.3825, 5.2672) (-74.2846, 5.3284) (-74.2723, 5.3896) knots 0 0 0 1 1 1
  line L1277 (-74.2723, 5.3896) -> (-74.3336, 5.4753)
  line L1278 (-74.3336, 5.4753) -> (-74.2723, 5.6345)
  spline S200 degree 2 poles (-74.2723, 5.6345) (-74.3825, 5.8672) (-74.5417, 5.8672) knots 0 0 0 1 1 1
  line L1279 (-74.5417, 5.8672) -> (-74.9091, 5.8672)
  spline S201 degree 2 poles (-74.9091, 5.8672) (-74.9703, 5.8059) (-74.9703, 5.7325) knots 0 0 0 1 1 1
  line L1280 (-74.9703, 5.7325) -> (-75.0193, 5.7325)
  spline S202 degree 2 poles (-75.0193, 5.7325) (-75.056, 5.5243) (-75.2152, 5.4753) knots 0 0 0 1 1 1
  spline S203 degree 2 poles (-75.2152, 5.4753) (-75.2519, 5.2794) (-75.4356, 5.2427) knots 0 0 0 1 1 1
  line L1281 (-75.4356, 5.2427) -> (-75.5703, 5.0223)
  line L1282 (-75.5703, 5.0223) -> (-75.607, 5.0223)
  spline S204 degree 2 poles (-75.607, 5.0223) (-75.656, 4.8508) (-75.7907, 4.8508) knots 0 0 0 1 1 1
  spline S205 degree 2 poles (-75.7907, 4.8508) (-75.9499, 4.8508) (-76.1336, 5.2917) (-76.1336, 5.3162) knots 0 0 0 1 2 2 2
  spline S206 degree 2 poles (-76.1336, 5.3162) (-76.1336, 5.3529) (-76.1091, 5.3896) knots 0 0 0 1 1 1
  spline S207 degree 2 poles (-76.1091, 5.3896) (-76.0233, 5.7202) (-75.6315, 5.9406) knots 0 0 0 1 1 1
  line L1283 (-75.6315, 5.9406) -> (-75.6315, 6.0019)
  spline S208 degree 2 poles (-75.6315, 6.0019) (-75.4601, 6.1733) (-75.2887, 6.2468) knots 0 0 0 1 1 1
  line L1284 (-75.2887, 6.2468) -> (-75.3621, 6.2468)
  spline S209 degree 2 poles (-75.3621, 6.2468) (-75.0315, 6.3202) (-74.9213, 6.859) (-74.5785, 6.859) knots 0 0 0 1 2 2 2
  line L1285 (-74.5785, 6.859) -> (-74.4927, 6.8223)
  line L1286 (-74.4927, 6.8223) -> (-74.2968, 6.9202)
  line L1287 (-74.2968, 6.9202) -> (-74.407, 6.9202)
  line L1288 (-74.407, 6.9202) -> (-74.2356, 7.0304)
  line L1289 (-74.2356, 7.0304) -> (-74.1866, 7.0059)
  line L1290 (-74.1866, 7.0059) -> (-74.0519, 7.1651)
  line L1291 (-74.0519, 7.1651) -> (-74.0152, 7.1406)
  spline S210 degree 2 poles (-74.0152, 7.1406) (-73.9295, 7.3611) (-73.5989, 7.3611) knots 0 0 0 1 1 1
  spline S211 degree 2 poles (-73.5989, 7.3611) (-73.5254, 7.3611) (-73.5254, 7.4223) knots 0 0 0 1 1 1
  line L1292 (-73.5254, 7.4223) -> (-73.5254, 7.4957)
  line L1293 (-73.5254, 7.4957) -> (-73.4642, 7.4957)
  line L1294 (-73.4642, 7.4957) -> (-73.4887, 7.5202)
  line L1295 (-73.4887, 7.5202) -> (-73.2438, 7.7039)
  spline S212 degree 2 poles (-73.2438, 7.7039) (-73.1213, 7.9121) (-72.8519, 7.9121) knots 0 0 0 1 1 1
  spline S213 degree 2 poles (-72.8519, 7.9121) (-72.6927, 7.9121) (-72.4356, 7.7284) (-72.4356, 7.6427) knots 0 0 0 1 2 2 2
  spline S214 degree 2 poles (-72.4356, 7.6427) (-72.4356, 7.5447) (-72.5458, 7.3611) knots 0 0 0 1 1 1
  line L1296 (-71.4438, 11.7937) -> (-71.4927, 11.7937)
  line L1297 (-71.4927, 11.7937) -> (-71.7744, 11.1937)
  line L1298 (-71.7744, 11.1937) -> (-71.7989, 11.2304)
  spline S215 degree 2 poles (-71.7989, 11.2304) (-71.7989, 11.1447) (-71.8723, 11.0835) knots 0 0 0 1 1 1
  line L1299 (-71.8723, 11.0835) -> (-71.8723, 11.059)
  spline S216 degree 2 poles (-71.8723, 11.059) (-72.0438, 10.7896) (-72.2887, 10.6672) knots 0 0 0 1 1 1
  line L1300 (-72.2887, 10.6672) -> (-72.3499, 10.6917)
  line L1301 (-72.3499, 10.6917) -> (-72.3499, 10.6427)
  spline S217 degree 2 poles (-72.3499, 10.6427) (-72.656, 10.6794) (-72.9744, 10.8508) (-73.1336, 11.2549) (-73.207, 11.4753) knots 0 0 0 1 2 3 3 3
  spline S218 degree 2 poles (-73.207, 11.4753) (-73.0968, 11.6345) (-73.0233, 11.659) knots 0 0 0 1 1 1
  line L1302 (-73.0233, 11.659) -> (-72.9621, 11.8672)
  line L1303 (-72.9621, 11.8672) -> (-72.7172, 12.0019)
  line L1304 (-72.7172, 12.0019) -> (-72.5703, 12.2957)
  line L1305 (-72.5703, 12.2957) -> (-72.3254, 12.4304)
  line L1306 (-72.3254, 12.4304) -> (-72.3254, 12.3937)
  line L1307 (-72.3254, 12.3937) -> (-72.1907, 12.3325)
  spline S219 degree 2 poles (-72.1907, 12.3325) (-72.1295, 12.357) (-72.0927, 12.3937) (-72.0315, 12.4549) (-71.7376, 12.5162) (-71.6642, 12.5651) knots 0 0 0 1 2 3 4 4 4
  line L1308 (-71.6642, 12.5651) -> (-71.5785, 12.6141)
  line L1309 (-71.5785, 12.6141) -> (-71.5172, 12.6141)
  line L1310 (-71.5172, 12.6141) -> (-71.407, 12.4304)
  line L1311 (-71.407, 12.4304) -> (-71.407, 12.1978)
  line L1312 (-71.407, 12.1978) -> (-71.3703, 11.9774)
  line L1313 (-71.3703, 11.9774) -> (-71.4438, 11.7937)
  spline S220 degree 2 poles (-65.7131, 10.2141) (-65.7131, 10.0549) (-65.9703, 9.6631) knots 0 0 0 1 1 1
  line L1314 (-65.9703, 9.6631) -> (-65.9703, 9.5162)
  line L1315 (-65.9703, 9.5162) -> (-66.1295, 9.1243)
  line L1316 (-66.1295, 9.1243) -> (-66.1295, 8.8794)
  line L1317 (-66.1295, 8.8794) -> (-66.3499, 8.3529)
  line L1318 (-66.3499, 8.3529) -> (-66.3499, 8.2794)
  spline S221 degree 2 poles (-66.3499, 8.2794) (-66.3499, 8.108) (-66.2397, 8.108) knots 0 0 0 1 1 1
  line L1319 (-66.2397, 8.108) -> (-65.9948, 8.1815)
  spline S222 degree 2 poles (-65.9948, 8.1815) (-65.7621, 8.0468) (-65.6029, 8.0468) knots 0 0 0 1 1 1
  line L1320 (-65.6029, 8.0468) -> (-65.2601, 8.0468)
  spline S223 degree 2 poles (-65.2601, 8.0468) (-64.7825, 8.1692) (-64.5499, 8.1692) knots 0 0 0 1 1 1
  spline S224 degree 2 poles (-64.5499, 8.1692) (-64.2682, 8.1692) (-63.9376, 8.1202) knots 0 0 0 1 1 1
  line L1321 (-63.9376, 8.1202) -> (-63.9376, 8.0713)
  line L1322 (-63.9376, 8.0713) -> (-63.656, 8.0468)
  line L1323 (-63.656, 8.0468) -> (-63.3989, 7.7284)
  line L1324 (-63.3989, 7.7284) -> (-63.6438, 7.4223)
  line L1325 (-63.6438, 7.4223) -> (-64.0846, 7.3611)
  line L1326 (-64.0846, 7.3611) -> (-64.5131, 7.1284)
  line L1327 (-64.5131, 7.1284) -> (-64.6846, 7.0917)
  spline S225 degree 2 poles (-64.6846, 7.0917) (-64.7703, 7.0794) (-64.9295, 6.9692) knots 0 0 0 1 1 1
  line L1328 (-64.9295, 6.9692) -> (-65.407, 7.0182)
  spline S226 degree 2 poles (-65.407, 7.0182) (-65.4438, 6.9447) (-65.8233, 6.9325) knots 0 0 0 1 1 1
  line L1329 (-65.8233, 6.9325) -> (-66.607, 6.908)
  spline S227 degree 2 poles (-66.607, 6.908) (-66.9376, 6.6631) (-67.0478, 6.5529) knots 0 0 0 1 1 1
  line L1330 (-67.0478, 6.5529) -> (-67.0233, 6.1611)
  line L1331 (-67.0233, 6.1611) -> (-67.1213, 5.9896)
  line L1332 (-67.1213, 5.9896) -> (-67.1825, 5.4264)
  line L1333 (-67.1825, 5.4264) -> (-67.3785, 5.1815)
  line L1334 (-67.3785, 5.1815) -> (-67.4029, 4.508)
  line L1335 (-67.4029, 4.508) -> (-67.5989, 4.41)
  line L1336 (-67.5989, 4.41) -> (-67.6233, 4.2141)
  line L1337 (-67.6233, 4.2141) -> (-67.5131, 3.8345)
  line L1338 (-67.5131, 3.8345) -> (-67.6601, 2.4264)
  line L1339 (-67.6601, 2.4264) -> (-67.3417, 1.2264)
  line L1340 (-67.3417, 1.2264) -> (-66.9866, 1.3733)
  spline S228 degree 2 poles (-66.9866, 1.3733) (-66.8887, 1.5815) (-66.607, 1.5815) knots 0 0 0 1 1 1
  line L1341 (-66.607, 1.5815) -> (-66.4601, 1.5815)